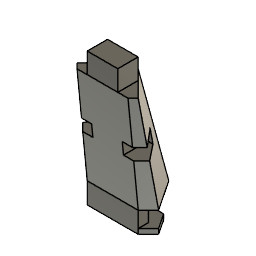
neck (Autodesk Fusion 360 design; units mm, degrees)
Autodesk Fusion 360 part; units mm, degrees
note: some values were not read from the file. Set by a fixed rule: which sketch regions a step uses.
sketch "Sketch1" plane through (0, 0, 0) normal (0, 0, 1) x (1, 0, 0)
  line L0 (50, 30) -> (20, 30)
  line L1 (0, 0) -> (20, 30)
  line L2 (50, 30) -> (70, 0)
  line L3 (0, 0) -> (10, -10)
  line L4 (10, -10) -> (60, -10)
  line L5 (60, -10) -> (70, 0)
  constraint horizontal L0
  constraint coincident L1.start L3.start
  constraint perpendicular L3 L5
ref_plane "WorkPlane1" through (0, 0, 100) normal (0, 0, 1) x (1, 0, 0)
sketch "Sketch2" plane through (0, 0, 100) normal (0, 0, 1) x (1, 0, 0)
  line L0 (30, 10) -> (40, 10)
  line L1 (60, -20) -> (10, -20)
  line L2 (30, 10) -> (5, -15)
  line L3 (5, -15) -> (10, -20)
  line L4 (40, 10) -> (65, -15)
  line L5 (65, -15) -> (60, -20)
  constraint horizontal L0
  constraint horizontal L1
  constraint perpendicular L2 L3
  constraint parallel L3 L4
  constraint perpendicular L4 L5
loft "Loft1" add profiles "Sketch1", "Sketch2" section 1 section 2 makes body 1
ref_plane "WorkPlane2" through (35, 10, 50) normal (0, 0, -1) x (-1, 0, 0)
sketch "Sketch3" plane through (0, 0, 50) normal (0, 0, -1) x (-1, 0, 0)
  line L0 (0.4452, 9.35) -> (-20, 9.35)
  line L1 (-20, 9.35) -> (-20, -30.9261)
  line L2 (-20, -30.9261) -> (0.4452, -30.9261)
  line L3 (0.4452, -30.9261) -> (0.4452, 9.35)
  line L4 (-69.0117, 9.35) -> (-50, 9.35)
  line L5 (-50, 9.35) -> (-50, -30.2583)
  line L6 (-50, -30.2583) -> (-69.0117, -30.2583)
  line L7 (-69.0117, -30.2583) -> (-69.0117, 9.35)
  constraint horizontal L0
  constraint vertical L1
  constraint horizontal L2
  constraint vertical L3
  constraint horizontal L4
  constraint vertical L5
  constraint horizontal L6
  constraint vertical L7
extrude "Extrude1" cut sketch "Sketch3" along normal blind -6 and the other way blind -6 bodies 1
ref_plane "WorkPlane3" through (35, 10, -15.5) normal (0, 0, -1) x (-1, 0, 0)
sketch "Sketch4" plane through (0, 0, -15.5) normal (0, 0, -1) x (-1, 0, 0)
  line L0 (-70, 0) -> (-60, 15)
  line L1 (0, 0) -> (-10, -10)
  line L2 (-10, -10) -> (-60, -10)
  line L3 (-60, -10) -> (-70, 0)
  line L4 (-10, 15) -> (0, 0)
  line L5 (-60, 15) -> (-10, 15)
  constraint coincident L1.start L4.end
  constraint horizontal L5
extrude "Extrude2" add sketch "Sketch4" along normal blind 5 separate body makes body 2
sketch "Sketch5" plane through (0, 0, 0) normal (0, 0, -1) x (1, 0, 0)
  line L0 (10, 10) -> (0, 0)
  line L1 (0, 0) -> (20, -30)
  line L2 (20, -30) -> (50, -30)
  line L3 (50, -30) -> (70, 0)
  line L4 (70, 0) -> (60, 10)
  line L5 (60, 10) -> (10, 10)
  line L6 (10, 10) -> (60, 10)
  line L7 (60, 10) -> (60, 0)
  line L8 (60, 0) -> (10, 0)
  line L9 (10, 0) -> (10, 10)
  constraint horizontal L6
  constraint vertical L7
  constraint horizontal L8
  constraint vertical L9
  constraint coincident L0.start L5.end
extrude "Extrude3" add sketch "Sketch5" along normal blind 20 contours L5 L6 L7 L8 L9 bodies 1 2
sketch "Sketch6" plane through (0, 0, 100) normal (0, 0, 1) x (-1, 0, 0)
  line L0 (-5, 15) -> (-10, 20)
  line L1 (-10, 20) -> (-60, 20)
  line L2 (-60, 20) -> (-65, 15)
  line L3 (-65, 15) -> (-40, -10)
  line L4 (-40, -10) -> (-30, -10)
  line L5 (-30, -10) -> (-5, 15)
  line L6 (-20, 0) -> (-50, 0)
  line L7 (-50, 0) -> (-50, 20)
  line L8 (-50, 20) -> (-20, 20)
  line L9 (-20, 20) -> (-20, 0)
  constraint horizontal L6
  constraint vertical L7
  constraint horizontal L8
  constraint vertical L9
  constraint coincident L1 L7.end
  constraint coincident L5 L6.start
extrude "Extrude4" add sketch "Sketch6" along normal blind 20 contours L1 L6 L7 L8 L9 bodies 1
